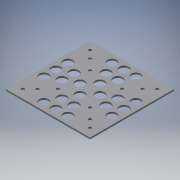
# Autodesk Inventor part: plate_mk2
Saved by Autodesk Inventor 2016 (Build 200138000, 138)
## iProperties
Created: 2015-09-10
Part Number: plate_mk2
Material: Generic
Document SubType Name: Modeling
Designer: Dima
Density: 1 g/cm^3
Appearance: Default
Author: Dima
Autodesk Inventor part; units mm, degrees
ref_plane "YZ Plane" through (0, 0, 0) normal (1, 0, 0) x (0, 1, 0)
ref_plane "XZ Plane" through (0, 0, 0) normal (0, 1, 0) x (-1, 0, 0)
ref_plane "XY Plane" through (0, 0, 0) normal (0, 0, 1) x (1, 0, 0)
sketch "Sketch1" plane through (0, 0, 0) normal (0, 1, 0) x (-1, 0, 0)
  line L0 (0, 0) -> (-80.01, 0)
  line L1 (-80.01, 0) -> (-80.01, -80.01)
  line L2 (-80.01, -80.01) -> (0, -80.01)
  line L3 (0, -80.01) -> (0, 0)
  dimension "d0" = 80.01
  dimension "d1" = 80.01
  constraints: 8 end point, 2 parallel, 1 horizontal, 1 perpendicular
  measures "d0" distance of L2.end L1.end
  measures "d1" distance of L1.end L0.end
extrude "Extrusion1" add sketch "Sketch1" along normal blind 1.524
sketch "Sketch2" plane through (0, 1.524, 0) normal (0, 1, 0) x (1, 0, 0)
  line L0 (0, 0) -> (80.01, 0) projected
  line L1 (80.01, 80.01) -> (0, 80.01) projected
  line L2 (0, 0) -> (8.001, 0)
  line L3 (8.001, 0) -> (8.001, 8.001)
  circle A0 centre (8.001, 8.001) radius 1.5
  line L4 (80.01, 0) -> (72.009, 0)
  line L5 (72.009, 0) -> (72.009, 8.001)
  line L6 (0, 80.01) -> (8.001, 80.01)
  line L7 (8.001, 80.01) -> (8.001, 72.009)
  line L8 (80.01, 80.01) -> (72.009, 80.01)
  line L9 (72.009, 80.01) -> (72.009, 72.009)
  circle A1 centre (8.001, 72.009) radius 1.4986
  circle A2 centre (72.009, 72.009) radius 1.4986
  circle A3 centre (72.009, 8.001) radius 1.4986
  line L10 (0, 0) -> (15.0114, 0)
  line L11 (15.0114, 0) -> (15.0114, 15.0114)
  line L12 (0, 80.01) -> (15.0114, 80.01)
  line L13 (15.0114, 80.01) -> (15.0114, 64.9986)
  line L14 (80.01, 80.01) -> (64.9986, 80.01)
  line L15 (64.9986, 80.01) -> (64.9986, 64.9986)
  line L16 (80.01, 0) -> (64.9986, 0)
  line L17 (64.9986, 0) -> (64.9986, 15.0114)
  circle A4 centre (15.0114, 15.0114) radius 1.4986
  circle A5 centre (15.0114, 64.9986) radius 1.4986
  circle A6 centre (64.9986, 64.9986) radius 1.4986
  circle A7 centre (64.9986, 15.0114) radius 1.4986
  dimension "d4" = 8.001
  dimension "d5" = 8.001
  dimension "d6" = 3
  dimension "d7" = 8.001
  dimension "d8" = 8.001
  dimension "d9" = 8.001
  dimension "d10" = 8.001
  dimension "d11" = 8.001
  dimension "d12" = 2.9972
  dimension "d13" = 2.9972
  dimension "d14" = 15.0114
  dimension "d15" = 15.0114
  dimension "d16" = 15.0114
  dimension "d17" = 15.0114
  dimension "d18" = 15.0114
  dimension "d19" = 15.0114
  dimension "d20" = 15.0114
  dimension "d21" = 15.0114
  dimension "d22" = 2.9972
  dimension "d23" = 2.9972
  dimension "d24" = 2.9972
  dimension "d25" = 2.9972
  constraints: 32 end point, 8 centre point, 8 coincident, 8 perpendicular, 8 point on line
  measures "d4" distance of L0.start L2.end
  measures "d5" distance of L2.end L3.end
  measures "d6" diameter of A0
  measures "d7" distance of L0.end L4.end
  measures "d8" distance of L4.end L5.end
  measures "d9" distance of L6.end L7.end
  measures "d10" distance of L1.start L8.end
  measures "d11" distance of L8.end L9.end
  measures "d12" diameter of A1
  measures "d13" diameter of A3
  measures "d14" distance of L0.start L10.end
  measures "d15" distance of L10.end L11.end
  measures "d16" distance of L1.end L12.end
  measures "d17" distance of L12.end L13.end
  measures "d18" distance of L1.start L14.end
  measures "d19" distance of L14.end L15.end
  measures "d20" distance of L0.end L16.end
  measures "d21" distance of L16.end L17.end
  measures "d22" diameter of A4
  measures "d23" diameter of A5
  measures "d24" diameter of A6
  measures "d25" diameter of A7
extrude "Extrusion2" cut sketch "Sketch2" against normal blind 1.524
sketch "Sketch3" plane through (0, 1.524, 0) normal (0, 1, 0) x (1, 0, 0)
  line L0 (0, 0) -> (80.01, 0) projected
  line L1 (80.01, 0) -> (80.01, 80.01) projected
  line L2 (80.01, 80.01) -> (0, 80.01) projected
  line L3 (0, 80.01) -> (0, 0) projected
  line L4 (40.005, 0) -> (40.005, 7.62)
  line L5 (0, 40.005) -> (7.62, 40.005)
  line L6 (40.005, 80.01) -> (40.005, 72.39)
  line L7 (80.01, 40.005) -> (72.39, 40.005)
  circle A0 centre (40.005, 72.39) radius 4.445
  circle A1 centre (40.005, 7.62) radius 4.445
  circle A2 centre (7.62, 40.005) radius 4.445
  circle A3 centre (72.39, 40.005) radius 4.445
  circle A4 centre (7.62, 28.575) radius 4.445
  circle A5 centre (72.39, 28.575) radius 4.445
  circle A6 centre (7.62, 51.435) radius 4.445
  circle A7 centre (72.39, 51.435) radius 4.445
  circle A8 centre (7.62, 40.005) radius 4.445
  circle A9 centre (72.39, 40.005) radius 4.445
  circle A10 centre (51.435, 72.39) radius 4.445
  circle A11 centre (51.435, 7.62) radius 4.445
  circle A12 centre (28.575, 72.39) radius 4.445
  circle A13 centre (28.575, 7.62) radius 4.445
  circle A14 centre (40.005, 72.39) radius 4.445
  circle A15 centre (40.005, 7.62) radius 4.445
  line L8 (19.05, 40.005) -> (19.05, 45.72)
  line L9 (19.05, 40.005) -> (19.05, 34.29)
  circle A16 centre (19.05, 45.72) radius 4.445
  circle A17 centre (19.05, 34.29) radius 4.445
  line L10 (7.62, 40.005) -> (19.05, 40.005)
  line L11 (19.05, 40.005) -> (30.48, 40.005)
  circle A18 centre (30.48, 40.005) radius 4.445
  line L12 (40.005, 72.39) -> (40.005, 60.96)
  line L13 (40.005, 60.96) -> (40.005, 49.53)
  line L14 (72.39, 40.005) -> (60.96, 40.005)
  line L15 (60.96, 40.005) -> (49.53, 40.005)
  line L16 (40.005, 7.62) -> (40.005, 19.05)
  line L17 (40.005, 19.05) -> (40.005, 30.48)
  line L18 (40.005, 19.05) -> (45.72, 19.05)
  line L19 (40.005, 19.05) -> (34.29, 19.05)
  line L20 (40.005, 60.96) -> (45.72, 60.96)
  line L21 (40.005, 60.96) -> (34.29, 60.96)
  line L22 (60.96, 40.005) -> (60.96, 45.72)
  line L23 (60.96, 40.005) -> (60.96, 34.29)
  circle A19 centre (40.005, 49.53) radius 4.445
  circle A20 centre (40.005, 30.48) radius 4.445
  circle A21 centre (49.53, 40.005) radius 4.445
  circle A22 centre (60.96, 45.72) radius 4.445
  circle A23 centre (60.96, 34.29) radius 4.445
  circle A24 centre (34.29, 60.96) radius 4.445
  circle A25 centre (45.72, 60.96) radius 4.445
  circle A26 centre (34.29, 19.05) radius 4.445
  circle A27 centre (45.72, 19.05) radius 4.445
  dimension "d28" = 7.62
  dimension "d29" = 7.62
  dimension "d30" = 7.62
  dimension "d31" = 7.62
  dimension "d32" = 8.89
  dimension "d33" = 8.89
  dimension "d34" = 8.89
  dimension "d35" = 8.89
  dimension "d45" = 11.43
  dimension "d52" = 11.43
  dimension "d66" = 11.43
  dimension "d69" = 11.43
  dimension "d74" = 11.43
  dimension "d77" = 11.43
  dimension "d111" = 5.715
  dimension "d112" = 5.715
  dimension "d113" = 8.89
  dimension "d114" = 8.89
  dimension "d115" = 11.43
  dimension "d116" = 8.89
  dimension "d117" = 11.43
  dimension "d118" = 11.43
  dimension "d119" = 11.43
  dimension "d120" = 11.43
  dimension "d121" = 11.43
  dimension "d122" = 5.715
  dimension "d123" = 5.715
  dimension "d124" = 5.715
  dimension "d125" = 5.715
  dimension "d126" = 5.715
  dimension "d127" = 5.715
  dimension "d128" = 8.89
  dimension "d129" = 8.89
  dimension "d130" = 8.89
  dimension "d131" = 8.89
  dimension "d132" = 8.89
  dimension "d133" = 8.89
  dimension "d134" = 8.89
  dimension "d135" = 8.89
  dimension "d136" = 8.89
  constraints: 40 end point, 28 centre point, 16 coincident, 8 horizontal, 7 vertical, 4 midpoint, 4 perpendicular, 4 point on line, 1 parallel, 24 other
  measures "d28" distance of L4.start L4.end
  measures "d29" distance of L5.start L5.end
  measures "d30" distance of L6.start L6.end
  measures "d31" distance of L7.start L7.end
  measures "d32" diameter of A0
  measures "d33" diameter of A1
  measures "d34" diameter of A2
  measures "d35" diameter of A3
  measures "d45" distance of A2.centre L8.start
  measures "d52" distance of A1.centre L16.end
  measures "d66" distance of A3.centre A5.centre
  measures "d69" distance of A3.centre A7.centre
  measures "d74" distance of A0.centre A10.centre
  measures "d77" distance of A0.centre A12.centre
  measures "d111" distance of L8.start L8.end
  measures "d112" distance of L8.start L9.end
  measures "d113" diameter of A16
  measures "d114" diameter of A17
  measures "d115" distance of L8.start L11.end
  measures "d116" diameter of A18
  measures "d117" distance of L12.start L12.end
  measures "d118" distance of L12.end L13.end
  measures "d119" distance of L14.start L14.end
  measures "d120" distance of L14.end L15.end
  measures "d121" distance of L16.end L17.end
  measures "d122" distance of L16.end L18.end
  measures "d123" distance of L16.end L19.end
  measures "d124" distance of L12.end L20.end
  measures "d125" distance of L12.end L21.end
  measures "d126" distance of L14.end L22.end
  measures "d127" distance of L14.end L23.end
  measures "d128" diameter of A19
  measures "d129" diameter of A20
  measures "d130" diameter of A21
  measures "d131" diameter of A22
  measures "d132" diameter of A23
  measures "d133" diameter of A24
  measures "d134" diameter of A25
  measures "d135" diameter of A26
  measures "d136" diameter of A27
sketch "Sketch4" plane through (0, 1.524, 0) normal (0, 1, 0) x (1, 0, 0)
  line L0 (0, 0) -> (80.01, 0) projected
  line L1 (0, 0) -> (24.7396, 0)
  line L2 (24.7396, 0) -> (24.7396, 24.7396)
  circle A0 centre (24.7396, 24.7396) radius 1.4986
  line L3 (80.01, 0) -> (55.2704, 0)
  line L4 (55.2704, 0) -> (55.2704, 24.7396)
  circle A1 centre (55.2704, 24.7396) radius 1.4986
  line L5 (80.01, 80.01) -> (0, 80.01) projected
  line L6 (0, 80.01) -> (24.7396, 80.01)
  line L7 (24.7396, 80.01) -> (24.7396, 55.2704)
  circle A2 centre (24.7396, 55.2704) radius 1.4986
  line L8 (80.01, 80.01) -> (55.2704, 80.01)
  line L9 (55.2704, 80.01) -> (55.2704, 55.2704)
  circle A3 centre (55.2704, 55.2704) radius 1.4986
  dimension "d98" = 24.7396
  dimension "d99" = 24.7396
  dimension "d100" = 2.9972
  dimension "d101" = 24.7396
  dimension "d102" = 24.7396
  dimension "d103" = 2.9972
  dimension "d104" = 24.7396
  dimension "d105" = 24.7396
  dimension "d106" = 2.9972
  dimension "d107" = 24.7396
  dimension "d108" = 24.7396
  constraints: 16 end point, 4 centre point, 4 coincident, 4 point on line, 3 perpendicular, 1 vertical
  measures "d98" distance of L0.start L1.end
  measures "d99" distance of L1.end L2.end
  measures "d100" diameter of A0
  measures "d101" distance of L0.end L3.end
  measures "d102" distance of L3.end L4.end
  measures "d103" diameter of A1
  measures "d104" distance of L5.end L6.end
  measures "d105" distance of L6.end L7.end
  measures "d106" diameter of A2
  measures "d107" distance of L5.start L8.end
  measures "d108" distance of L8.end L9.end
extrude "Extrusion4" cut sketch "Sketch4" against normal blind 25.4
extrude "Extrusion5" cut sketch "Sketch3" against normal blind 25.4 contours A26 | A20 | A27 | A1 L16 L4 | L4 L16 A1 | A23 | A21 | A22 | A3 L14 L7 | L7 L14 A3 | A25 | A19 | A24 | A0 L12 L6 | L6 L12 A0 | A16 | A18 | A17 | A2 L10 L5 | L5 L10 A2 | A4 | A5 | A6 | A7 | A10 | A11 | A12 | A13
body "Solid1"
